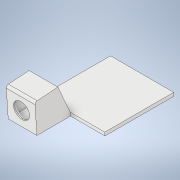
# Autodesk Inventor part: Airunit_aufnahme
Saved by Autodesk Inventor 2020 (Build 240168000, 168)
## iProperties
Part Number: Airunit_aufnahme
Material: GEDA Polyamid
Document SubType Name: Modeling
Designer: Admin
Mass: 32.8262 g
Surface Area: 124.605 cm^2
Volume: 28.7949 cm^3
Density: 1.14 g/cm^3
Appearance: GEDA Polyamid A
Gewicht: 0,033 kg
G_L: 0
G_H: 0
G_B: 0
InventorVersion: 2019.4
VAULT_Status: in Bearbeitung
Revision: -
Max. Breite: 0
Max. Höhe: 0
Max. Länge: 0
Max. Abmessungen: 0 x 0 x 0
Volumen: 28794,908
Author: Admin
Autodesk Inventor part; units mm, degrees
note: some values were not read from the file. Left out: dimensions or parameters whose unit could not be read.
ref_plane "YZ Plane" through (0, 0, 0) normal (1, 0, 0) x (0, 1, 0)
ref_plane "XZ Plane" through (0, 0, 0) normal (0, 1, 0) x (-1, 0, 0)
ref_plane "XY Plane" through (0, 0, 0) normal (0, 0, 1) x (1, 0, 0)
sketch "Skizze1" plane through (0, 0, 0) normal (1, 0, 0) x (0, 1, 0)
  line L0 (60, -3) -> (60, 0)
  line L1 (60, 0) -> (0, 0)
  line L2 (0, 0) -> (-10.8137, 24.3352)
  line L3 (-29, -3) -> (-30.8137, 22.9367)
  line L4 (-30.8137, 22.9367) -> (-10.8137, 24.3352)
  line L5 (-29, -3) -> (60, -3)
  dimension "d52" = 3
  dimension "d56" = 26
  dimension "d57" = 20
  dimension "d88" = 60
  dimension "d89" = 94
  dimension "d90" = 29
  constraints: 12 end point, 2 perpendicular, 1 coincident, 1 parallel, 1 vertical
  measures "d52" distance of L0.start L0.end
  measures "d56" distance of L3.start L3.end
  measures "d57" horizontal distance of L3.end L2.end
  measures "d88" distance of L0.end L1.end
  measures "d89" angle of L5 L3
  measures "d90" horizontal distance of L3.start point (0, 0)
extrude "Extrusion1" add sketch "Skizze1" along normal mid plane 50
sketch "Skizze10" plane through (-25, -30.8137, 22.9367) normal (0, -0.0698, 0.9976) x (1, 0, 0)
  line L0 (50, 29.1386) -> (0, 29.1386) projected
  line L1 (25, 29.1386) -> (25, 0) construction
  line L2 (0, 0) -> (50, 0) projected
  line L3 (25, 0) -> (50, 0)
  line L4 (50, 0) -> (50, 29.1386)
  line L5 (50, 29.1386) -> (25, 29.1386)
  line L6 (25, 29.1386) -> (25, 0)
  constraints: 10 end point, 2 midpoint, 2 parallel, 1 horizontal, 1 perpendicular
extrude "Extrusion8" cut sketch "Skizze10" against normal through all
sketch "Skizze17" plane through (-25, -30.8137, 22.9367) normal (0, -0.9976, -0.0698) x (1, 0, 0)
  circle A0 centre (12.5, -13) radius 7
  line L0 (25, -26) -> (25, 0) projected
  line L1 (25, 0) -> (0, 0) projected
  point P0 (25, -25.0302)
  point P1 (25, -13)
  point P2 (12.5, 0)
  dimension "d91" = 14
  constraints: 2 midpoint, 1 centre point, 1 horizontal alignment, 1 vertical alignment
  measures "d91" diameter of A0
extrude "Extrusion13" cut sketch "Skizze17" against normal blind 3
sketch "Skizze18" plane through (-12.5, -26.9141, 10.1776) normal (0, -0.9976, -0.0698) x (1, 0, 0)
  line L0 (10.25, -11) -> (-10.25, -11)
  line L1 (-10.25, -11) -> (-10.25, 11)
  line L2 (-10.25, 11) -> (10.25, 11)
  line L3 (10.25, 11) -> (10.25, -11)
  line L4 (10.25, -11) -> (-10.25, 11) construction
  line L5 (-10.25, -11) -> (10.25, 11) construction
  line L6 (12.5, -13) -> (12.5, 13) projected
  line L7 (12.5, 13) -> (-12.5, 13) projected
  point P0 (12.5, -12.0302)
  point P1 (0, 0)
  point P2 (0, 0)
  point P3 (12.5, 0)
  point P4 (0, 0)
  point P5 (0, 13)
  dimension "d94" = 20.5
  dimension "d95" = 22
  constraints: 12 end point, 6 midpoint, 2 parallel, 1 horizontal, 1 horizontal alignment, 1 perpendicular, 1 vertical alignment
  measures "d94" distance of L1.end L2.end
  measures "d95" distance of L0.end L1.end
extrude "Extrusion14" cut sketch "Skizze18" against normal up to next
fillet "Rundung18" radius 2 1 edges at (-19.5, -26.9141, 10.1776)
fillet "Rundung19" radius 2 1 edges at (-12.5, -30.8137, 22.9367)
sketch "Skizze19" plane through (25, 0, 0) normal (1, 0, 0) x (0, 0, -1)
  line L0 (0, 0) -> (3, 0.2098) projected
  line L1 (3, 0.2098) -> (3, 60) projected
  line L2 (3, 60) -> (0, 60) projected
  line L3 (0, 60) -> (0, 0) projected
extrude "Extrusion15" add sketch "Skizze19" along normal blind 5
equation "\"G_L\" = 0"
equation "\"G_H\" = 0"
equation "\"G_B\" = 0"
